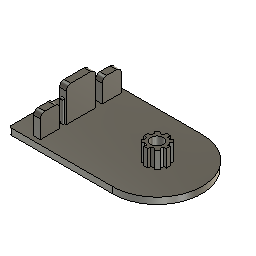
ROULEAUcover (Autodesk Fusion 360 design; units mm, degrees)
Autodesk Fusion 360 part; units mm, degrees
note: some values were not read from the file. Set by a fixed rule: which sketch regions a step uses.
sketch "Sketch1" plane through (0, 0, 0) normal (0, 0, 1) x (1, 0, 0) in component "body"
  line L0 (33, -20) -> (-33, -20)
  line L1 (-33, -20) -> (-33, 20)
  line L2 (-33, 20) -> (33, 20)
  line L3 (33, 20) -> (33, -20)
  line L4 (33, -20) -> (-33, 20) construction
  line L5 (-33, -20) -> (33, 20) construction
  circle A0 centre (13, 0) radius 2.75
  line L6 (1.75, 0) -> (22.5, 0)
  circle A1 centre (13, 0) radius 4
  line L7 (18, -0.9) -> (8, -0.9)
  line L8 (8, -0.9) -> (8, 0.9)
  line L9 (8, 0.9) -> (18, 0.9)
  line L10 (18, 0.9) -> (18, -0.9)
  line L11 (18, -0.9) -> (8, 0.9) construction
  line L12 (8, -0.9) -> (18, 0.9) construction
  line L13 (17.1719, 2.8991) -> (10.1009, -4.1719)
  line L14 (15.8991, 4.1719) -> (17.1719, 2.8991)
  line L15 (8.8281, -2.8991) -> (15.8991, 4.1719)
  line L16 (10.1009, -4.1719) -> (8.8281, -2.8991)
  line L17 (13.9, 5) -> (13.9, -5)
  line L18 (12.1, 5) -> (13.9, 5)
  line L19 (12.1, -5) -> (12.1, 5)
  line L20 (13.9, -5) -> (12.1, -5)
  line L21 (10.1009, 4.1719) -> (17.1719, -2.8991)
  line L22 (8.8281, 2.8991) -> (10.1009, 4.1719)
  line L23 (15.8991, -4.1719) -> (8.8281, 2.8991)
  line L24 (17.1719, -2.8991) -> (15.8991, -4.1719)
  line L25 (-21, -18) -> (-24, -18)
  line L26 (-24, -18) -> (-24, -9.5)
  line L27 (-24, -9.5) -> (-21, -9.5)
  line L28 (-21, -9.5) -> (-21, -18)
  line L29 (-21, 9.5) -> (-21, 18)
  line L30 (-24, 9.5) -> (-21, 9.5)
  line L31 (-24, 18) -> (-24, 9.5)
  line L32 (-21, 18) -> (-24, 18)
  line L33 (-24, -6.5) -> (-21, -6.5)
  line L34 (-21, -6.5) -> (-21, 6.5)
  line L35 (-21, 6.5) -> (-24, 6.5)
  line L36 (-24, 6.5) -> (-24, -6.5)
  line L37 (-24, -6.5) -> (-21, 6.5) construction
  line L38 (-21, -6.5) -> (-24, 6.5) construction
  circle A2 centre (-22.5, 6.5) radius 0.75
  circle A3 centre (-22.5, -6.5) radius 0.75
  point P0 (13, 0)
  point P1 (-22.5, 0)
  dimension "d1" = 66
  dimension "d2" = 40
  dimension "d3" = 5.5
  dimension "d4" = 20
  dimension "d5" = 8
  dimension "d6" = 10
  dimension "d7" = 1.8
  dimension "d13" = 135
  dimension "d20" = 3
  dimension "d21" = 8.5
  dimension "d22" = 9
  dimension "d23" = 2
  dimension "d24" = 3
  dimension "d25" = 13
  dimension "d26" = 9
  dimension "d33" = 1.5
  dimension "d34" = 1.5
  constraint horizontal L0
  constraint perpendicular L0 L1
  constraint parallel L0 L2
  constraint parallel L1 L3
  constraint coincident L4 origin
  constraint coincident L5 origin
  constraint coincident P0 L6
  constraint concentric A0 A1
  constraint horizontal L7
  constraint perpendicular L7 L8
  constraint parallel L7 L9
  constraint parallel L8 L10
  constraint coincident L11 P0
  constraint coincident L12 P0
  constraint coincident P0 A0.centre
  constraint horizontal L25
  constraint vertical L26
  constraint horizontal L27
  constraint vertical L28
  constraint symmetric L6 L25.start L29.end
  constraint symmetric L6 L25.end L31.start
  constraint symmetric L6 L26.end L30.start
  constraint symmetric L6 L27.end L29.start
  constraint horizontal L33
  constraint perpendicular L33 L34
  constraint parallel L33 L35
  constraint parallel L34 L36
  constraint coincident L37 P1
  constraint coincident L38 P1
  constraint coincident L6 P1
  constraint midpoint L35 A2.centre
  constraint midpoint L33 A3.centre
  measures "d1" distance of L1.end L2.end
  measures "d2" distance of L0.end L1.end
  measures "d3" diameter of A0
  measures "d4" distance of L3 P0
  measures "d5" diameter of A1
  measures "d6" distance of L8.end L9.end
  measures "d7" distance of L7.end L8.end
  measures "d20" distance of L25.start L25.end
  measures "d21" distance of L25.start L27.end
  measures "d22" distance of L1 L26
  measures "d23" distance of L0 L25
  measures "d24" distance of L34.end L35.end
  measures "d25" distance of L33.end L34.end
  measures "d26" distance of L1 L36
  measures "d33" diameter of A2
  measures "d34" diameter of A3
extrude "Extrude3" add sketch "Sketch1" along normal blind 3 contours L0 L1 L2 L3 | A0 L6 L9 L13 | A0 L6 A1 L7 | A0 L6 A1 L9 | A0 L6 L7 L21 | A0 L9 L13 | A0 A1 L9 L13 | A0 A1 L7 L21 | A0 L7 L21 | L6 A1 L9 L10 | L6 A1 L7 L10 | L6 L13 L17 | L9 L13 L17 L21 | L7 L13 L17 L21 | L6 L17 L21 | A0 L9 L13 L15 L17 | A0 A1 L13 L15 | A0 A1 L21 L23 | A0 L7 L17 L21 L23 | L6 L7 L13 L17 L19 L23 | L6 L9 L15 L17 L19 L21 | L7 L13 L17 | L9 L17 L21 | A0 L15 L17 | A0 A1 L15 L17 | A1 L13 L14 L15 | L9 L15 L17 L21 | A0 A1 L17 L23 | A0 L17 L23 | A1 L21 L23 L24 | L7 L13 L17 L23 | L6 L19 L23 | L6 L15 L19 | L7 L13 L23 | L9 L15 L21 | A0 L15 L17 L19 L21 | A0 A1 L17 L19 | A0 A1 L17 L19 | A0 L13 L17 L19 L23 | A0 L6 L7 L15 | L7 L15 L19 L23 | L9 L15 L19 L23 | A0 L6 L9 L23 | L7 L19 L23 | L9 L15 L19 | L7 L13 L19 L23 | L9 L15 L19 L21 | A0 L19 L21 | A0 A1 L19 L21 | A1 L17 L18 L19 | A0 A1 L13 L19 | A0 L13 L19 | A1 L17 L19 L20 | A0 L6 A1 L9 | A0 L6 A1 L7 | A0 L7 L15 | A0 L7 L13 L15 L19 | A0 L9 L19 L21 L23 | A0 L9 L23 | A0 A1 L21 L23 | A0 A1 L13 L15 | A0 A1 L9 L23 | A0 A1 L7 L15 | L6 A1 L7 L8 | L6 A1 L8 L9 | A1 L21 L22 L23 | A1 L13 L15 L16 | L25 L26 L27 L28 | L29 L30 L31 L32 | L33 L34 L35 L36 A2 A3 | L33 A3 | L33 A3 | L35 A2 | L35 A2 makes body 1 in component "body"
extrude "Extrude1" add sketch "Sketch1" along normal blind 10.5 separate body contours A0 L6 A1 L7 | A0 L6 A1 L9 | A0 A1 L9 L13 | A0 A1 L7 L21 | A0 A1 L13 L15 | A0 A1 L21 L23 | A0 A1 L15 L17 | A0 A1 L17 L23 | A0 A1 L17 L19 | A0 A1 L17 L19 | A0 A1 L19 L21 | A0 A1 L13 L19 | A0 L6 A1 L9 | A0 L6 A1 L7 | A0 A1 L21 L23 | A0 A1 L13 L15 | A0 A1 L9 L23 | A0 A1 L7 L15 makes body 2 in component "body"
extrude "Extrude2" add sketch "Sketch1" along normal blind 10.5 contours L6 A1 L9 L10 | L6 A1 L7 L10 | A1 L13 L14 L15 | A1 L21 L23 L24 | A1 L17 L18 L19 | A1 L17 L19 L20 | L6 A1 L7 L8 | L6 A1 L8 L9 | A1 L21 L22 L23 | A1 L13 L15 L16 bodies 2 1 in component "body"
fillet "Fillet1" radius 20 2 edges at (33, -20, 1.5) (33, 20, 1.5) on bodies 2 in component "body"
fillet "Fillet1" radius 1 2 edges at (-33, -20, 1.5) (-33, 20, 1.5) on bodies 2 in component "body"
extrude "Extrude4" add sketch "Sketch1" along normal blind 13 contours L25 L26 L27 L28 | L29 L30 L31 L32 bodies 2 in component "body"
extrude "Extrude5" add sketch "Sketch1" along normal blind 18 contours L33 L34 L35 L36 A2 A3 | L33 A3 | L35 A2 picked at (-22.3167, -6.33) picked at (-22.3854, 5.9564) bodies 2 in component "body"
extrude "Extrude6" add sketch "Sketch1" along normal blind 13 contours L33 A3 | L33 A3 | L35 A2 | L35 A2 bodies 2 in component "body"
fillet "Fillet2" radius 2 6 edges at (-22.5, 18, 13) (-22.5, 6.5, 18) (-22.5, -6.5, 18) (-22.5, -9.5, 13) (-22.5, -18, 13) (-22.5, 9.5, 13) on bodies 2 in component "body"
fillet "Fillet2" radius 0.7 2 edges at (-22.5, 7.25, 13) (-22.5, -7.25, 13) on bodies 2 in component "body"
chamfer "Chamfer1" distance 0.2 distance2 3 6 edges at (-9.5, 20, 0) (33, 0, 0) (-9.5, -20, 0) (-32.7071, -19.7071, 0) (-33, 0, 0) (-32.7071, 19.7071, 0) measured on face at (-1.9974, 6.6667, 0) measured on face at (33, 0.0013, 1) measured on face at (-1.9974, 6.6667, 0) measured on face at (-32.0952, -19.9955, 1) measured on face at (-1.9974, 6.6667, 0) measured on face at (-32.3718, 19.9284, 1) on bodies 2 in component "body"
component "body" placed x (1, 0, 0) y (0, 1, 0) z (0, 0, 1) at (0, 0, 0)
